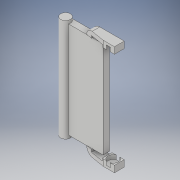
# Autodesk Inventor part: 20_Rect_Aperture_door_hinge
Saved by Autodesk Inventor 2019 (Build 230136000, 136)
## iProperties
Created: 2020-03-03
Part Number: 20_Rect_Aperture_door_hinge
Material: Generic
Document SubType Name: Modeling
Designer: marsikovabarbora
Density: 1 g/cm^3
Appearance: Default
Author: marsikovabarbora
Autodesk Inventor part; units mm, degrees
ref_plane "YZ Plane" through (0, 0, 0) normal (1, 0, 0) x (0, 1, 0)
ref_plane "XZ Plane" through (0, 0, 0) normal (0, 1, 0) x (-1, 0, 0)
ref_plane "XY Plane" through (0, 0, 0) normal (0, 0, 1) x (1, 0, 0)
sketch "Sketch1" plane through (0, 0, 0) normal (0, 0, 1) x (1, 0, 0)
  line L0 (-8.4, 0) -> (8.4, 0) construction
  line L1 (0, -20.65) -> (0, 20.65) construction
  line L2 (6, -14.75) -> (-6, -14.75)
  line L3 (-6, -14.75) -> (-6, 14.75)
  line L4 (-6, 14.75) -> (6, 14.75)
  line L5 (6, 14.75) -> (6, -14.75)
  line L6 (6, -14.75) -> (-6, 14.75) construction
  line L7 (-6, -14.75) -> (6, 14.75) construction
  point P0 (0, 0)
  dimension "d0" = 12
  dimension "d1" = 29.5
  constraints: 12 end point, 2 midpoint, 2 parallel, 1 horizontal, 1 perpendicular
  measures "d0" distance of L3.end L4.end
  measures "d1" distance of L2.end L3.end
extrude "Extrusion1" add sketch "Sketch1" along normal blind 2
sketch "Sketch3" plane through (-6, 14.75, 2) normal (0, 1, 0) x (1, 0, 0)
  line L0 (0, 2) -> (12, 2) construction
  line L1 (0, 2) -> (0, 0) construction
  line L2 (12, 0) -> (0, 0) construction
  circle A0 centre (0, 0.5) radius 1.5
  line L3 (12, 2) -> (12, 0) projected
  point P0 (6, 2)
  dimension "d7" = 3
  constraints: 1 horizontal, 1 vertical alignment, 2 other
extrude "Extrusion3" add sketch "Sketch3" against normal up to surface (29.5 mm away)
sketch "Sketch5" plane through (6, 14.75, 2) normal (0, 1, 0) x (1, 0, 0)
  arc A0 (-12, 2) -> (-10.5858, 0) centre (-12, 0.5) ccw construction
  line L0 (0, 0) -> (-10.5858, 0) construction
  line L1 (0, 2) -> (0, 0) construction
  line L2 (-12, 2) -> (0, 2) construction
  circle A1 centre (-12, 0.5) radius 1.5
  point P0 (-6, 2)
  constraints: 1 centre point, 1 coincident, 1 concentric
extrude "Extrusion5" add sketch "Sketch5" along normal blind 1
mirror "Mirror3" about plane through (0, 0, 0) normal (0, 1, 0) of "Extrusion5"
sketch "Sketch6" plane through (0, 0, 2) normal (0, 0, 1) x (1, 0, 0)
  line L0 (-4.5858, 14.75) -> (-4.5858, -14.75) construction
  line L1 (-4.5858, -14.75) -> (6, -14.75) construction
  line L2 (6, -14.75) -> (6, 14.75) construction
  line L3 (6, 14.75) -> (-4.5858, 14.75) construction
  line L4 (-9.1, 0) -> (12.6, 0) construction
  line L5 (-6, 14.75) -> (6, 14.75) projected
  line L6 (1, 14.75) -> (1, 16.75)
  line L7 (1, 16.75) -> (10.5, 16.75)
  line L8 (2.75, 15.5) -> (2.75, 14.75)
  line L9 (1, 14.75) -> (2.75, 14.75)
  line L10 (2.75, 15.5) -> (6.75, 15.5)
  line L11 (6.75, 15.5) -> (6.75, 14.75)
  line L12 (6.75, 14.75) -> (10.5, 14.75)
  line L13 (10.5, 16.75) -> (10.5, 14.75)
  line L14 (6, 14.75) -> (-4.5858, 14.75) projected
  line L15 (1, -14.75) -> (1, -16.75)
  line L16 (1, -16.75) -> (10.5, -16.75)
  line L17 (2.75, -15.5) -> (2.75, -14.75)
  line L18 (1, -14.75) -> (2.75, -14.75)
  line L19 (2.75, -15.5) -> (6.75, -15.5)
  line L20 (6.75, -15.5) -> (6.75, -14.75)
  line L21 (6.75, -14.75) -> (10.5, -14.75)
  line L22 (10.5, -16.75) -> (10.5, -14.75)
  line L23 (0, 14.75) -> (0, 17.3845) construction
  point P0 (0, 0)
  dimension "d14" = 2
  dimension "d15" = 0.75
  dimension "d16" = 0.75
  dimension "d17" = 1.75
  dimension "d18" = 4.5
  dimension "d40" = 1
  constraints: 34 end point, 8 symmetric about line, 4 perpendicular, 2 collinear, 2 point on line, 2 vertical, 1 horizontal
  measures "d14" distance of L6.start L6.end
  measures "d15" distance of L8.start L8.end
  measures "d16" distance between parallel lines of L2 L11
  measures "d17" distance between parallel lines of L6 L8
  measures "d18" distance between parallel lines of L2 L13
  measures "d40" distance between parallel lines of L23 L6
extrude "Extrusion6" add sketch "Sketch6" against normal up to surface (2 mm away)
sketch "Skizze9" plane through (0, 0, 2) normal (0, 0, 1) x (1, 0, 0)
  line L0 (-4.5858, 14.75) -> (-4.5858, -14.75) construction
  line L1 (-4.5858, -14.75) -> (1, -14.75) construction
  line L2 (1, -14.75) -> (1, -16.75) construction
  line L3 (1, -16.75) -> (10.5, -16.75) construction
  line L4 (10.5, -16.75) -> (10.5, -14.75) construction
  line L5 (10.5, -14.75) -> (6.75, -14.75) construction
  line L6 (6.75, -14.75) -> (6.75, -15.5) construction
  line L7 (6.75, -15.5) -> (2.75, -15.5) construction
  line L8 (2.75, -15.5) -> (2.75, -14.75) construction
  line L9 (2.75, -14.75) -> (6, -14.75) construction
  line L10 (6, -14.75) -> (6, 14.75) construction
  line L11 (6, 14.75) -> (2.75, 14.75) construction
  line L12 (2.75, 14.75) -> (2.75, 15.5) construction
  line L13 (2.75, 15.5) -> (6.75, 15.5) construction
  line L14 (6.75, 15.5) -> (6.75, 14.75) construction
  line L15 (6.75, 14.75) -> (10.5, 14.75) construction
  line L16 (10.5, 14.75) -> (10.5, 16.75) construction
  line L17 (10.5, 16.75) -> (1, 16.75) construction
  line L18 (1, 16.75) -> (1, 14.75) construction
  line L19 (1, 14.75) -> (-4.5858, 14.75) construction
  line L20 (1, 14.75) -> (-4.5858, 14.75) projected
  line L21 (1, 16.75) -> (1, 14.75) projected
  line L22 (1, 14.75) -> (1, 16.75)
  line L23 (1, 16.75) -> (10.5, 16.75)
  line L24 (10.5, 14.75) -> (10.5, 16.75) projected
  line L25 (10.5, 16.75) -> (10.5, 14.75)
  line L26 (10.5, 14.75) -> (6.75, 14.75)
  line L27 (6.75, 15.5) -> (6.75, 14.75) projected
  line L28 (6.75, 14.75) -> (6.75, 15.5)
  line L29 (6.75, 15.5) -> (2.75, 15.5) projected
  line L30 (6.75, 15.5) -> (2.75, 15.5)
  line L31 (2.75, 14.75) -> (2.75, 15.5) projected
  line L32 (2.75, 15.5) -> (2.75, 14.75)
  line L33 (2.75, 14.75) -> (1, 14.75)
  line L34 (1, -16.75) -> (1, -14.75) projected
  line L35 (1, -14.75) -> (1, -16.75)
  line L36 (1, -16.75) -> (10.5, -16.75)
  line L37 (10.5, -16.75) -> (10.5, -14.75) projected
  line L38 (10.5, -16.75) -> (10.5, -14.75)
  line L39 (10.5, -14.75) -> (6.75, -14.75)
  line L40 (6.75, -14.75) -> (6.75, -15.5) projected
  line L41 (6.75, -14.75) -> (6.75, -15.5)
  line L42 (6.75, -15.5) -> (2.75, -15.5)
  line L43 (2.75, -15.5) -> (2.75, -14.75)
  line L44 (2.75, -14.75) -> (1, -14.75)
  point P0 (0, 0)
  constraints: 32 end point, 7 collinear, 7 perpendicular, 2 vertical
extrude "Extrusion9" add sketch "Skizze9" along normal blind 1
sketch "Skizze10" plane through (0, 0, 0) normal (0, 1, 0) x (-1, 0, 0)
  line L0 (-10.5, 0) -> (-1, 0) construction
  line L1 (-10.5, 0) -> (-10.5, 3) construction
  line L2 (-1, 3) -> (-10.5, 3) construction
  line L3 (-1, 0) -> (-1, 3) construction
  line L4 (-10.5, 0) -> (-6.75, 0) construction
  line L5 (-10.5, 0) -> (-10.5, 3) construction
  line L6 (-6.75, 3) -> (-10.5, 3) construction
  line L7 (-6.75, 0) -> (-6.75, 3) construction
  line L8 (-6.75, 1.5) -> (-10.5, 1.5) construction
  line L9 (-10.5, 3) -> (-1, 3) construction
  line L10 (-10.5, 0) -> (-6.75, 0) construction
  line L11 (-8.625, 0) -> (-8.625, 3) construction
  line L12 (-6.75, 3) -> (-10.5, 3) construction
  circle A0 centre (-8.625, 1.5) radius 1.6
  point P0 (0, 0)
  dimension "d32" = 3.2
  constraints: 5 midpoint, 4 end point, 1 centre point
  measures "d32" diameter of A0
extrude "Extrusion10" cut sketch "Skizze10" along normal mid plane 32
chamfer "Fase1" distance 6 distance2 1 1 edges at (1, 15.75, 3) measured on face at (6.5227, 16.5, 3)
chamfer "Fase2" distance 6 distance2 1 1 edges at (1, -15.75, 3) measured on face at (6.5227, -16.5, 3)
fillet "Rundung1" radius 2 2 edges at (1, 16.75, 1) (1, -16.75, 1)
body "Solid1"
